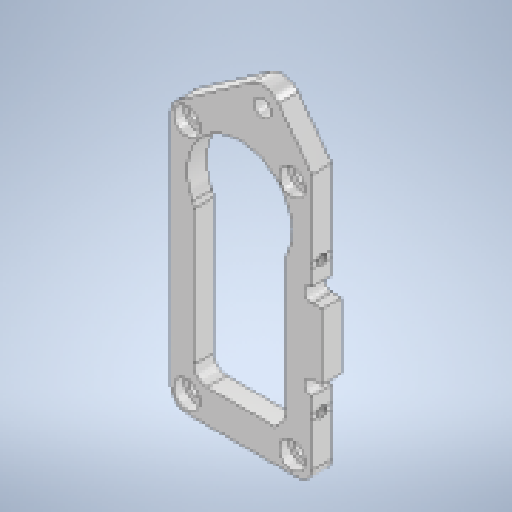
# Autodesk Inventor part: kosi_pti
Saved by Autodesk Inventor 2025.1 (Build 291241000, 241)
## iProperties
Created: 2024-09-01
Part Number: kosi_pti
Material: アルミニウム 2014-T4
Document SubType Name: Modeling
Designer: right
Density: 2.8 g/cm^3
Appearance: サテン
Mass: 3.87879 g
Surface Area: 18.6489 cm^2
Volume: 1.38528 cm^3
Author: right
Autodesk Inventor part; units mm, degrees
ref_plane "YZ Plane" through (0, 0, 0) normal (1, 0, 0) x (0, 1, 0)
ref_plane "XZ Plane" through (0, 0, 0) normal (0, 1, 0) x (-1, 0, 0)
ref_plane "XY Plane" through (0, 0, 0) normal (0, 0, 1) x (1, 0, 0)
sketch "スケッチ1" plane through (0, 0, 0) normal (0, 0, 1) x (1, 0, 0)
  circle A0 centre (20.7151, -6.426) radius 1 projected
  circle A1 centre (4.7151, -6.426) radius 1 projected
  circle A2 centre (20.7151, -6.426) radius 1.1
  circle A3 centre (20.7151, -6.426) radius 2.5
  circle A4 centre (4.7151, -6.426) radius 1.1
  circle A5 centre (4.7151, -6.426) radius 2.5
  circle A6 centre (16.2151, 1.074) radius 1.3
  circle A7 centre (16.2151, 1.074) radius 5
  line L0 (22.2151, -3.926) -> (3.2151, -3.926) projected
  line L1 (20.7151, -8.926) -> (4.7151, -8.926)
  line L2 (21.059, 2.3137) -> (23.137, -5.8062)
  line L3 (12.7668, 4.6947) -> (2.991, -4.6157)
  circle A8 centre (16.2151, 1.074) radius 3
  line L4 (18.8716, 2.4679) -> (22.9288, -5.2644)
  line L5 (14.4859, 3.5255) -> (3.2741, -4.3831)
  circle A9 centre (20.7151, -42.426) radius 1.8 projected
  circle A10 centre (20.7151, -42.426) radius 1.1
  circle A11 centre (20.7151, -42.426) radius 2.5
  line L6 (20.7151, -3.926) -> (23.7151, -3.926)
  line L7 (23.7151, -3.926) -> (23.7151, -44.926)
  line L8 (23.7151, -44.926) -> (20.7151, -44.926)
  line L9 (18.2151, -6.426) -> (18.2151, -42.426)
  line L10 (18.6151, 2.874) -> (23.7151, -3.926)
  circle A12 centre (4.7151, -42.426) radius 1 projected
  circle A13 centre (4.7151, -42.426) radius 1.1
  circle A14 centre (4.7151, -42.426) radius 2.5
  line L11 (20.7151, -44.926) -> (4.7151, -44.926)
  line L12 (20.7151, -39.926) -> (4.7151, -39.926)
  circle A15 centre (12.7151, -12.926) radius 8 projected
  point P0 (0, 0)
  point P1 (3.9221, -3.926)
  point P2 (3.7151, -3.926)
  point P3 (22.2266, -3.926)
  point P4 (18.2151, -39.926)
  point P5 (18.2151, -8.926)
  point P6 (19.4225, -8.5659)
  point P7 (18.3559, -7.2531)
  point P8 (18.2151, -7.1165)
  point P9 (18.2151, -18.7355)
  point P10 (5.7869, -8.926)
  point P11 (19.6433, -8.926)
  dimension "d0" = 2.2
  dimension "d1" = 5
  dimension "d2" = 2.2
  dimension "d3" = 5
  dimension "d4" = 2.6
  dimension "d5" = 10
  dimension "d8" = 13
  dimension "d9" = 6
  dimension "d10" = 2.2
  dimension "d11" = 5
  dimension "d12" = 3
  dimension "d43" = 2.2
  constraints: 24 end point, 18 point on circle, 18 tangent, 11 centre point, 9 coincident, 2 horizontal, 1 collinear, 1 concentric, 1 equal radius, 1 perpendicular
  measures "d0" diameter of A2
  measures "d1" diameter of A3
  measures "d2" diameter of A4
  measures "d3" diameter of A5
  measures "d4" diameter of A6
  measures "d5" diameter of A7
  measures "d8" horizontal distance of L0.end A7.centre
  measures "d9" diameter of A8
  measures "d10" diameter of A10
  measures "d11" diameter of A11
  measures "d12" distance of L7.end L8.end
  measures "d43" diameter of A13
extrude "押し出し1" add sketch "スケッチ1" along normal blind 3 contours A3 A15 | A3 L2 L6 L7 L8 A11 L12 L9 A15 L1 | A3 L4 L6 L2 | L1 A15 A3 | A3 L0 L6 L4 | L6 L4 A7 L10 L2 | L2 L10 L6 | L0 A7 L4 L6 | A3 L9 A15 A5 L0 | A15 L9 A3 | L0 L5 A7 | A7 L5 A8 L4 | L4 A8 L10 A7 | L1 A5 A15 | A5 A15 | A5 L5 L0 | A8 | L11 A14 L12 L9 A11 | A11 | L12 A11 L9 | A14 | A9 picked at (22.7275, -6.6114) picked at (3.1651, -5.1285)
sketch "スケッチ3" plane through (0, 0, 3) normal (0, 0, 1) x (1, 0, 0)
  circle A0 centre (20.7151, -6.426) radius 1.1 projected
  circle A1 centre (20.7151, -6.426) radius 2
  circle A2 centre (4.7151, -6.426) radius 1.1 projected
  circle A3 centre (4.7151, -6.426) radius 2
  circle A4 centre (20.7151, -42.426) radius 1.1 projected
  circle A5 centre (20.7151, -42.426) radius 2
  circle A6 centre (4.7151, -42.426) radius 1.1 projected
  circle A7 centre (4.7151, -42.426) radius 2
  point P0 (0, 0)
  dimension "d13" = 4
  dimension "d14" = 4
  dimension "d15" = 4
  dimension "d44" = 4
  constraints: 4 centre point, 4 coincident
  measures "d13" diameter of A1
  measures "d14" diameter of A3
  measures "d15" diameter of A5
  measures "d44" diameter of A7
extrude "押し出し2" cut sketch "スケッチ3" against normal blind 1.5 contours A0 | A1 | A3 | A4 | A5 | A7
sketch "スケッチ4" plane through (0, 0, 3) normal (0, 0, 1) x (1, 0, 0)
  line L0 (15.2865, -30.6046) -> (19.1437, -30.6046) projected
  line L1 (19.1437, -30.6046) -> (19.1437, -24.2474) projected
  line L2 (19.1437, -24.2474) -> (15.2865, -24.2474) projected
  circle A0 centre (20.7151, -42.426) radius 2 projected
  circle A1 centre (4.7151, -6.426) radius 2 projected
  circle A2 centre (20.7151, -6.426) radius 2 projected
  arc A3 (3.2741, -4.3831) -> (4.7151, -8.926) centre (4.7151, -6.426) ccw projected
  line L3 (4.7151, -8.926) -> (5.7869, -8.926) projected
  arc A4 (18.2151, -18.7355) -> (5.7869, -8.926) centre (12.7151, -12.926) ccw projected
  line L4 (18.2151, -18.7355) -> (18.2151, -39.926) projected
  line L5 (23.7151, -44.926) -> (23.7151, -3.926) projected
  line L6 (23.7151, -3.926) -> (18.6151, 2.874) projected
  arc A5 (18.6151, 2.874) -> (14.4859, 3.5255) centre (16.2151, 1.074) ccw projected
  line L7 (14.4859, 3.5255) -> (3.2741, -4.3831) projected
  circle A6 centre (16.2151, 1.074) radius 1.3 projected
  line L8 (15.2865, -23.7474) -> (19.6437, -23.7474)
  line L9 (19.6437, -23.7474) -> (19.6437, -31.1046)
  line L10 (19.6437, -31.1046) -> (15.2865, -31.1046)
  line L11 (18.2151, -39.926) -> (4.7151, -39.926) projected
  arc A7 (4.7151, -39.926) -> (4.7151, -44.926) centre (4.7151, -42.426) ccw projected
  line L12 (4.7151, -44.926) -> (23.7151, -44.926) projected
  point P0 (0, 0)
  point P1 (18.2151, -31.1046)
  point P2 (18.2151, -23.7474)
  dimension "d18" = 0.5
  constraints: 6 end point, 2 other
  measures "d18" distance between parallel lines of L1 L9
extrude "押し出し3" cut sketch "スケッチ4" against normal through all contours L4 L2 L1 L0 | L0 L1 L2 L4 L8 L9 L10
fillet "フィレット1" radius 2 4 edges at (18.2151, -31.1046, 1.5) (19.6437, -31.1046, 1.5) (18.2151, -23.7474, 1.5) (19.6437, -23.7474, 1.5)
sketch "スケッチ5" plane through (23.7151, -44.926, 0) normal (1, 0, 0) x (0, 0, -1)
  line L0 (0, 0) -> (-3, 0) projected
  line L1 (0, 41) -> (-3, 41) projected
  point P0 (0, 44.926)
  point P1 (-1.5, 9)
  point P2 (-1.5, 29)
  point P3 (-1.5, 0)
  point P4 (-1.5, 41)
  point P5 (-1.5, 0)
  dimension "d22" = 12
  dimension "d42" = 20
  constraints: 3 midpoint, 2 vertical alignment
  measures "d22" distance of point (-1.5, 41) point (-1.5, 29)
  measures "d42" distance of point (-1.5, 29) point (-1.5, 9)
hole "穴1" at (23.7151, -15.926, 1.5) at (23.7151, -35.926, 1.5) direction (-1, 0, 0) diameter 1.567 depth 6.3 tip angle 118 thread size "M2x0.4" class "6H" standard "ISO Metric profile"
sketch "スケッチ6" plane through (0, 0, 3) normal (0, 0, 1) x (1, 0, 0)
  line L0 (23.7151, -15.1425) -> (23.7151, -16.7095) projected
  line L1 (23.7151, -35.1425) -> (23.7151, -36.7095) projected
  circle A0 centre (24.7151, -15.926) radius 1.1
  circle A1 centre (24.7151, -35.926) radius 1.1
  point P0 (0, 0)
  point P1 (23.7151, -15.926)
  point P2 (23.7151, -35.926)
  dimension "d31" = 2.2
  dimension "d32" = 1
  dimension "d33" = 2.2
  constraints: 2 centre point, 2 horizontal alignment, 2 midpoint, 1 vertical alignment
  measures "d31" diameter of A0
  measures "d32" distance from line of L0 A0.centre
  measures "d33" diameter of A1
extrude "押し出し4" cut sketch "スケッチ6" against normal through all
sketch "スケッチ7" plane through (0, 0, 3) normal (0, 0, 1) x (1, 0, 0)
  line L0 (18.2151, -9.426) -> (18.2151, -39.426)
  line L1 (18.2151, -39.426) -> (19.7151, -39.426)
  line L2 (19.7151, -39.426) -> (19.7151, -9.426)
  line L3 (19.7151, -9.426) -> (18.2151, -9.426)
  line L4 (23.7151, -35.4677) -> (23.7151, -16.3843) projected
  circle A0 centre (20.7151, -42.426) radius 1.1 projected
  circle A1 centre (20.7151, -6.426) radius 1.1 projected
  point P0 (0, 0)
  point P1 (18.2151, -22.6001)
  dimension "d36" = 4
  dimension "d37" = 3
  dimension "d38" = 3
  constraints: 8 end point, 3 perpendicular, 1 point on line, 1 vertical
  measures "d36" distance between parallel lines of L2 L4
  measures "d37" distance from line of A0.centre L1
  measures "d38" distance from line of A1.centre L3
extrude "押し出し5" cut sketch "スケッチ7" against normal through all contours L3 L2 L1 L0
fillet "フィレット2" radius 2 3 edges at (19.7151, -39.426, 1.5) (18.2151, -39.426, 1.5) (23.7151, -44.926, 1.5)
sketch "スケッチ10" plane through (0, 0, 3) normal (0, 0, 1) x (1, 0, 0)
  arc A0 (3.2741, -4.3831) -> (4.7151, -8.926) centre (4.7151, -6.426) ccw projected
  line L0 (2.2151, -6.426) -> (2.2151, -42.426)
  arc A1 (4.7151, -39.926) -> (4.7151, -44.926) centre (4.7151, -42.426) ccw projected
  line L1 (5.7869, -8.926) -> (5.7869, -39.926)
  line L2 (18.2151, -39.926) -> (4.7151, -39.926) projected
  line L3 (4.7151, -8.926) -> (5.7869, -8.926) projected
  arc A2 (20.6403, -14.0176) -> (19.0909, -8.094) centre (12.7151, -12.926) ccw projected
  circle A3 centre (12.7151, -12.926) radius 8
  point P0 (0, 0)
  point P1 (5.7869, -16.926)
  constraints: 4 end point, 2 point on circle, 2 tangent, 1 coincident, 1 point on line, 1 vertical, 3 other
extrude "押し出し8" add sketch "スケッチ10" against normal up to surface (3 mm away) contours A0 L3 A3 L1 L2 A1 L0
fillet "フィレット4" radius 2 3 edges at (5.7869, -39.926, 1.5) (5.7869, -16.926, 1.5) (19.7151, -16.799, 1.5)
sketch "スケッチ11" plane through (23.7151, -35.4677, 0) normal (1, 0, 0) x (0, 0, -1)
  line L0 (0, 0) -> (0, 19.0835) projected
  line L1 (-3, 0) -> (-3, 19.0835) projected
  line L2 (0, 14.5417) -> (-3, 14.5417)
  line L3 (-3, 14.5417) -> (-3, 4.5417)
  line L4 (-3, 4.5417) -> (0, 4.5417)
  line L5 (0, 4.5417) -> (0, 14.5417)
  point P0 (0, 35.4677)
  point P1 (0, 9.5417)
  point P2 (0, 9.5417)
  point P3 (0, 4.5417)
  dimension "d59" = 10
  constraints: 8 end point, 2 midpoint, 2 parallel, 2 point on line, 1 coincident, 1 horizontal, 1 perpendicular
  measures "d59" distance between parallel lines of L2 L4
extrude "押し出し9" add sketch "スケッチ11" along normal blind 1.5
sketch "スケッチ12" plane through (0, 0, 3) normal (0, 0, 1) x (1, 0, 0)
  line L0 (23.7151, -20.926) -> (23.7151, -16.3843) projected
  circle A0 centre (23.7151, -19.826) radius 1.1
  line L1 (25.2151, -20.926) -> (25.2151, -30.926) construction
  line L2 (25.2151, -25.926) -> (19.7151, -25.926) construction
  line L3 (19.7151, -37.4895) -> (19.7151, -17.2849) construction
  circle A1 centre (23.7151, -32.026) radius 1.1
  point P0 (0, 0)
  point P1 (23.7151, -18.726)
  dimension "d62" = 2.2
  constraints: 2 end point, 2 point on line, 1 centre point, 1 horizontal, 1 midpoint, 1 symmetric about line, 4 other
extrude "押し出し10" cut sketch "スケッチ12" against normal through all contours A0 L0 | A1 picked at (22.9998, -20.0845)
sketch "スケッチ13" plane through (2.2151, -42.426, 3) normal (-1, 0, 0) x (0, 0, 1)
  circle A0 centre (-1.5, 6.5) radius 0.7835 projected
  arc A1 (-0.8645, 26.9583) -> (-2.1355, 26.9583) centre (-1.5, 26.5) ccw construction
  point P0 (-3, 42.426)
  constraints: 2 coincident
hole "穴2" at (2.2151, -15.926, 1.5) at (2.2151, -35.926, 1.5) direction (1, 0, 0) diameter 1.567 end through all thread size "M2x0.4" class "6H" standard "ISO Metric profile"
sketch "スケッチ14" plane through (0, 0, 3) normal (0, 0, 1) x (1, 0, 0)
  circle A0 centre (1.2151, -35.926) radius 1.1
  circle A1 centre (1.2151, -15.926) radius 1.1
  line L0 (2.2151, -36.7095) -> (2.2151, -35.1425) projected
  line L1 (2.2151, -16.7095) -> (2.2151, -15.1425) construction
  point P0 (0, 0)
  point P1 (2.2151, -35.926)
  point P2 (2.2151, -15.926)
  dimension "d72" = 2.2
  dimension "d73" = 2.2
  dimension "d74" = 1
  dimension "d75" = 1
  constraints: 2 centre point, 2 horizontal alignment, 2 midpoint
  measures "d72" diameter of A0
  measures "d73" diameter of A1
  measures "d74" distance from line of L0 A0.centre
  measures "d75" distance from line of L1 A1.centre
extrude "押し出し11" cut sketch "スケッチ14" against normal through all
sketch "スケッチ15" plane through (2.2151, -35.4677, 3) normal (-1, 0, 0) x (0, 0, 1)
  line L0 (-3, 14.5417) -> (0, 14.5417) projected
  line L1 (-3, 4.5417) -> (-3, 14.5417) projected
  line L2 (0, 14.5417) -> (0, 4.5417) projected
  line L3 (0, 4.5417) -> (-3, 4.5417) projected
  point P0 (-3, 35.4677)
extrude "押し出し12" add sketch "スケッチ15" along normal blind 1.5
sketch "スケッチ16" plane through (0, 0, 3) normal (0, 0, 1) x (1, 0, 0)
  line L0 (2.2151, -20.926) -> (2.2151, -16.3843) projected
  circle A0 centre (2.2151, -19.826) radius 1.1
  line L1 (2.2151, -35.4677) -> (2.2151, -30.926) projected
  circle A1 centre (2.2151, -32.026) radius 1.1
  point P0 (0, 0)
  point P1 (2.2151, -33.126)
  point P2 (2.2151, -18.726)
  dimension "d80" = 2.2
  constraints: 2 point on line, 6 other
extrude "押し出し13" cut sketch "スケッチ16" against normal through all contours L0 A0 | L1 A1 picked at (2.6069, -19.5393) picked at (2.812, -31.7266)
sketch "スケッチ8" plane through (0, 0, 3) normal (0, 0, 1) x (1, 0, 0)
  circle A0 centre (13.2151, -51.926) radius 3
  circle A1 centre (13.2151, -51.926) radius 1.6
  line L0 (4.7151, -44.926) -> (21.7151, -44.926) projected
  arc A2 (21.7151, -44.926) -> (23.7151, -42.926) centre (21.7151, -42.926) ccw projected
  line L1 (23.2753, -44.1773) -> (15.5554, -53.803)
  line L2 (13.2151, -44.926) -> (13.2151, -39.926) construction
  line L3 (18.2151, -39.926) -> (4.7151, -39.926) construction
  line L4 (3.1549, -44.1773) -> (10.8748, -53.803)
  arc A3 (4.7151, -39.926) -> (4.7151, -44.926) centre (4.7151, -42.426) ccw projected
  point P0 (0, 0)
  point P1 (3.5047, -44.6134)
  dimension "d45" = 6
  dimension "d46" = 3.2
  dimension "d47" = 7
  constraints: 6 end point, 2 midpoint, 2 symmetric about line, 1 centre point, 1 coincident, 1 point on circle, 1 point on line, 1 tangent, 1 vertical, 1 vertical alignment, 4 other
  measures "d46" diameter of A1
  measures "d47" distance of point (13.215, -44.926) point (13.215, -51.926)
sketch "スケッチ9" plane through (0, 0, 3) normal (0, 0, 1) x (1, 0, 0)
  circle A0 centre (13.2151, -51.926) radius 1.6 projected
  arc A1 (18.8775, -39.117) -> (18.2151, -39.926) centre (20.0399, -40.7445) ccw projected
  line L0 (18.2151, -39.926) -> (4.7151, -39.926) projected
  arc A2 (4.7151, -39.926) -> (3.5047, -44.6134) centre (4.7151, -42.426) ccw projected
  line L1 (3.5047, -44.6134) -> (10.8748, -53.803) projected
  arc A3 (10.8748, -53.803) -> (15.5554, -53.803) centre (13.2151, -51.926) ccw projected
  line L2 (15.5554, -53.803) -> (23.2753, -44.1773) projected
  arc A4 (23.2753, -44.1773) -> (23.7151, -42.926) centre (21.7151, -42.926) ccw projected
  line L3 (23.7151, -42.926) -> (23.7151, -23.3843) projected
  arc A5 (23.7151, -22.4677) -> (23.7151, -23.3843) centre (24.7151, -22.926) ccw projected
  line L4 (23.7151, -22.4677) -> (23.7151, -12.3843) projected
  arc A6 (23.7151, -11.4677) -> (23.7151, -12.3843) centre (24.7151, -11.926) ccw projected
  line L5 (23.7151, -11.4677) -> (23.7151, -3.926) projected
  line L6 (23.7151, -3.926) -> (18.6151, 2.874) projected
  arc A7 (18.6151, 2.874) -> (14.4859, 3.5255) centre (16.2151, 1.074) ccw projected
  line L7 (14.4859, 3.5255) -> (3.2741, -4.3831) projected
  arc A8 (3.2741, -4.3831) -> (4.7151, -8.926) centre (4.7151, -6.426) ccw projected
  line L8 (4.7151, -8.926) -> (5.7869, -8.926) projected
  arc A9 (19.7151, -16.799) -> (5.7869, -8.926) centre (12.7151, -12.926) ccw projected
  line L9 (19.7151, -16.799) -> (19.7151, -37.4895) projected
  arc A10 (18.8775, -39.117) -> (19.7151, -37.4895) centre (17.7151, -37.4895) ccw projected
  circle A11 centre (4.7151, -6.426) radius 2 projected
  circle A12 centre (20.7151, -6.426) radius 2 projected
  circle A13 centre (20.7151, -42.426) radius 2 projected
  circle A14 centre (4.7151, -42.426) radius 2 projected
  circle A15 centre (16.2151, 1.074) radius 1.3 projected
  line L10 (20.5121, -44.426) -> (15.7648, -50.3452)
  circle A16 centre (13.2151, -51.926) radius 3
  line L11 (15.5554, -53.803) -> (23.2753, -44.1773) projected
  line L12 (10.6654, -50.3452) -> (5.9181, -44.426)
  line L13 (3.5047, -44.6134) -> (10.8748, -53.803) projected
  line L14 (20.5121, -44.426) -> (5.9181, -44.426)
  point P0 (0, 0)
  dimension "d50" = 2
  dimension "d51" = 2
  dimension "d52" = 2
  constraints: 6 end point, 3 point on circle, 2 parallel, 1 centre point, 1 coincident, 1 horizontal
  measures "d50" distance from line of A13.centre L14
  measures "d51" distance between parallel lines of L2 L10
  measures "d52" distance between parallel lines of L13 L12
equation "\"d1\" = d3"
equation "\"d11\" = d1"
equation "\"d38\" = d37"
equation "\"d52\" = d51"
